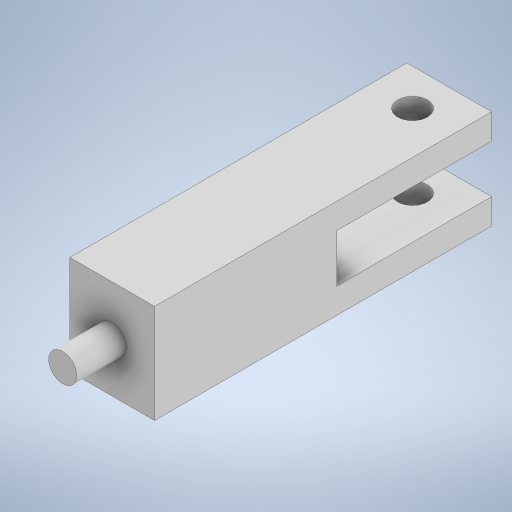
# Autodesk Inventor part: Link2
Saved by Autodesk Inventor 2024 (Build 280153000, 153)
## iProperties
Created: 2023-12-17
Part Number: Link2
Material: Generic
Document SubType Name: Modeling
Designer: pratikhya
Density: 1 g/cm^3
Appearance: Default
Author: pratikhya
Autodesk Inventor part; units mm, degrees
ref_plane "YZ Plane" through (0, 0, 0) normal (1, 0, 0) x (0, 1, 0)
ref_plane "XZ Plane" through (0, 0, 0) normal (0, 1, 0) x (-1, 0, 0)
ref_plane "XY Plane" through (0, 0, 0) normal (0, 0, 1) x (1, 0, 0)
sketch "Sketch1" plane through (0, 0, 0) normal (1, 0, 0) x (0, 1, 0)
  point P0 (0, 0)
sketch "Sketch2" plane through (0, 0, 0) normal (1, 0, 0) x (0, 1, 0)
  line L0 (3.1716, 6.9287) -> (-3.8284, 6.9287)
  line L1 (3.1716, 6.9287) -> (3.1716, -16.9242)
  line L2 (3.1716, -16.9242) -> (1.3716, -16.9242)
  line L3 (1.3716, -16.9242) -> (1.3716, -5.9694)
  line L4 (1.3716, -5.9694) -> (-2.0284, -5.9694)
  line L5 (-2.0284, -5.9694) -> (-2.0284, -16.9242)
  line L6 (-2.0284, -16.9242) -> (-3.8284, -16.9242)
  line L7 (-3.8284, -16.9242) -> (-3.8284, 6.9287)
  point P0 (0, 0)
  dimension "d0" = 7
  dimension "d2" = 1.8
  dimension "d6" = 3.4
  dimension "d8" = 1.8
  constraints: 16 end point, 3 horizontal, 3 perpendicular, 1 vertical
  measures "d0" distance of L0.start L0.end
  measures "d2" distance of L1.end L2.end
  measures "d6" distance of L3.end L4.end
  measures "d8" distance of L5.end L6.end
extrude "Extrusion1" add sketch "Sketch2" along normal blind 6
sketch "Sketch3" plane through (0, 3.1716, 6.9287) normal (0, 1, 0) x (1, 0, 0)
  line L0 (0, 23.8529) -> (6, 23.8529) projected
  circle A0 centre (3, 32.5) radius 1
  point P0 (0, 6.9287)
  dimension "d12" = 2
  constraints: 1 centre point
  measures "d12" diameter of A0
extrude "Extrusion2" cut sketch "Sketch3" against normal blind 9.875
sketch "Sketch5" plane through (0, 3.1716, 6.9287) normal (0, 1, 0) x (1, 0, 0)
  point P0 (0, 6.9287)
sketch "Sketch7" plane through (0, -3.8284, 6.9287) normal (0, 0, 1) x (1, 0, 0)
  line L0 (0, 1.8) -> (0, 5.2) projected
  line L1 (0, 3.5) -> (6, 3.5)
  line L2 (6, 1.8) -> (6, 5.2) projected
  line L3 (0, 0) -> (6, 0) projected
  line L4 (3, 0) -> (3, 7)
  line L5 (2, 7) -> (4, 7) projected
  circle A0 centre (3, 3.5) radius 1
  point P0 (0, 3.8284)
  dimension "d21" = 2
  constraints: 5 midpoint, 4 end point, 1 centre point
  measures "d21" diameter of A0
extrude "Extrusion5" add sketch "Sketch7" along normal blind 3.5
sketch "Sketch8" plane through (0, 3.1716, 6.9287) normal (0, 1, 0) x (1, 0, 0)
  line L0 (0, 0) -> (0, 23.8529) projected
  line L1 (0, 21.256) -> (5.958, 21.256)
  line L2 (5.958, 21.256) -> (3, 23.8529)
  line L3 (0, 23.8529) -> (6, 23.8529) projected
  line L4 (3, 23.8529) -> (3, 17.8866)
  circle A0 centre (3, 21.256) radius 1.0543
  point P0 (0, 6.9287)
  constraints: 6 end point, 3 point on line, 1 centre point, 1 horizontal, 1 midpoint, 1 vertical
extrude "Extrusion6" cut sketch "Sketch8" against normal blind 39.2125 contours A0 L4 L1 | L1 L4 A0 | L4 A0 L1 | L1 A0 L4
body "Solid1"
